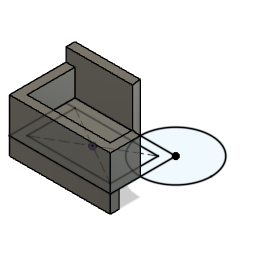
LD2540 Support (Autodesk Fusion 360 design; units mm, degrees)
Autodesk Fusion 360 part; units mm, degrees
sketch "Sketch1" plane through (0, 0, 0) normal (0, 1, 0) x (1, 0, 0)
  line L0 (-4.7, 2.7) -> (4.7, 2.7)
  line L1 (4.7, 2.7) -> (4.7, -2.7)
  line L2 (4.7, -2.7) -> (-4.7, -2.7)
  line L3 (-4.7, -2.7) -> (-4.7, 2.7)
  line L4 (-4.7, 2.7) -> (4.7, -2.7) construction
  line L5 (4.7, 2.7) -> (-4.7, -2.7) construction
  line L6 (-5.7, 3.7) -> (5.7, 3.7)
  line L7 (5.7, 3.7) -> (5.7, -3.7)
  line L8 (5.7, -3.7) -> (-5.7, -3.7)
  line L9 (-5.7, -3.7) -> (-5.7, 3.7)
  circle A0 centre (5.7, 3.7) radius 4
  line L10 (-4.7, 2.7) -> (-5.7, 2.7)
  dimension "d1" = 9.4
  dimension "d2" = 5.4
  dimension "d3" = -1
  dimension "d12" = 8
  constraint horizontal L0
  constraint perpendicular L0 L1
  constraint parallel L0 L2
  constraint parallel L1 L3
  constraint coincident L4 origin
  constraint coincident L5 origin
  constraint coincident L6.end L7.start
  constraint coincident L9 L10.end
  constraint perpendicular L9 L10
  measures "d1" distance of L1.end L2.end
  measures "d2" distance of L0.end L1.end
  measures "d12" diameter of A0
extrude "Extrude1" add sketch "Sketch1" along normal blind 4 contours L0 L6 L9 A0 L10 | L1 L2 L3 L7 L8 L9 A0 L10 | L0 L1 L6 L7 A0
extrude "Extrude2" add sketch "Sketch1" along normal blind 1 contours L0 L1 L2 L3 A0 | L0 L1 A0
sketch "Sketch2" plane through (0, 0, 0) normal (0, 1, 0) x (1, 0, 0)
  line L0 (-5.7, -3.7) -> (5.7, -3.7)
  line L1 (5.7, -3.7) -> (5.7, -2.7)
  line L2 (5.7, -2.7) -> (-5.7, -2.7)
  line L3 (-5.7, -2.7) -> (-5.7, -3.7)
  point P0 (-5.7, -3.7)
  dimension "d8" = 1
  dimension "d11" = 11.4
  constraint horizontal L0
  constraint vertical L1
  constraint horizontal L2
  constraint vertical L3
  constraint coincident P0 L0.start
  measures "d8" distance of P0 L2.end
  measures "d11" distance of P0 L0.end
extrude "Extrude3" add sketch "Sketch2" against normal blind 2
extrude "Extrude4" cut sketch "Sketch1" along normal blind 5 contours L0 L1 L6 L7 A0 | L0 L1 A0
extrude "Extrude5" add sketch "Sketch1" along normal blind 5.5 contours L0 L6 L9 A0 L10
named bodies: "LD2540 Support"
